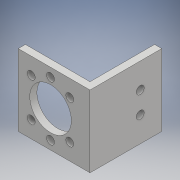
# Autodesk Inventor part: LBent_PScrew
Saved by Autodesk Inventor 2017 (Build 210142000, 142)
## iProperties
Created: 2017-03-12
Part Number: LBent_PScrew
Material: Generic
Document SubType Name: Modeling
Designer: umr
Density: 1 g/cm^3
Appearance: Default
Author: umr
Autodesk Inventor part; units mm, degrees
ref_plane "YZ Plane" through (0, 0, 0) normal (1, 0, 0) x (0, 1, 0)
ref_plane "XZ Plane" through (0, 0, 0) normal (0, 1, 0) x (-1, 0, 0)
ref_plane "XY Plane" through (0, 0, 0) normal (0, 0, 1) x (1, 0, 0)
sketch "Sketch1" plane through (0, 0, 0) normal (0, 0, 1) x (1, 0, 0)
  line L0 (0, 0) -> (-5, 0)
  line L1 (-5, 5) -> (-5, 50)
  line L2 (-5, 50) -> (0, 50)
  line L3 (0, 50) -> (0, 0)
  line L4 (0, 0) -> (-50, 0)
  line L5 (-50, 0) -> (-50, 5)
  line L6 (-50, 5) -> (-5, 5)
  line L7 (0, 5) -> (0, 0)
  dimension "d0" = 5
  dimension "d1" = 50
  dimension "d2" = 50
  dimension "d3" = 5
  constraints: 16 end point, 4 parallel, 2 horizontal, 2 perpendicular
  measures "d0" distance of L1.end L2.end
  measures "d1" distance of L0.end L1.end
  measures "d2" distance of L5.end L7.start
  measures "d3" distance of L4.end L5.end
extrude "Extrusion1" add sketch "Sketch1" along normal blind 50
sketch "Sketch3" plane through (-50, 5, 0) normal (0, 1, 0) x (1, 0, 0)
  circle A0 centre (22.5, -25) radius 14.5
  line L0 (45, 0) -> (0, 0) projected
  line L1 (0, 0) -> (0, -50) projected
  line L2 (45, -50) -> (0, -50) projected
  line L3 (45, 0) -> (45, -50) projected
  line L4 (22.5, -25) -> (0, -25)
  line L5 (22.5, -25) -> (22.5, 0)
  line L6 (45, 0) -> (0, 0) projected
  circle A1 centre (35.935, -38.435) radius 2.75
  circle A2 centre (9.065, -38.435) radius 2.75
  circle A3 centre (22.5, -44) radius 2.75
  circle A4 centre (35.935, -11.565) radius 2.75
  circle A5 centre (9.065, -11.565) radius 2.75
  circle A6 centre (22.5, -6) radius 2.75
  point P0 (50, 0)
  dimension "d44" = 29
  dimension "d45" = 45
  dimension "d46" = 22.5
  dimension "d47" = 25
  dimension "d48" = 5.5
  dimension "d49" = 13.435
  dimension "d50" = 13.435
  dimension "d51" = 5.5
  dimension "d52" = 13.435
  dimension "d53" = 13.435
  dimension "d54" = 5.5
  dimension "d55" = 19
  dimension "d56" = 0
  constraints: 7 centre point, 4 end point, 3 symmetric about line, 2 midpoint, 1 perpendicular, 3 other
  measures "d44" diameter of A0
  measures "d45" distance of L0.start L0.end
  measures "d46" distance from line of L1 L4.start
  measures "d47" distance from line of L0 L4.start
  measures "d48" diameter of A1
  measures "d49" horizontal distance of L4.start A1.centre
  measures "d50" distance from line of L5 A1.centre
  measures "d51" diameter of A2
  measures "d52" distance from line of L4 A2.centre
  measures "d53" distance from line of L5 A2.centre
  measures "d54" diameter of A3
  measures "d55" distance of L4.start A3.centre
  measures "d56" horizontal distance of L4.start A3.centre
extrude "Extrusion2" cut sketch "Sketch3" against normal blind 20 contours A0 L4 L5 | L5 L4 A0 | A6 L5 | L5 A6 | A1 | A2 | A3 | A4 | A5
sketch "Sketch4" plane through (-5, 5, 0) normal (-1, 0, 0) x (0, 0, 1)
  circle A0 centre (17.5, 30) radius 2.75
  line L0 (0, 45) -> (0, 0) projected
  line L1 (0, 45) -> (50, 45) projected
  circle A1 centre (32.5, 30) radius 2.75
  point P0 (0, -5)
  dimension "d59" = 5.5
  dimension "d61" = 17.5
  dimension "d64" = 45
  dimension "d65" = 15
  dimension "d68" = 5.5
  dimension "d69" = 15
  dimension "d70" = 15
  dimension "d71" = 50
  constraints: 2 centre point
  measures "d59" diameter of A0
  measures "d61" distance from line of L0 A0.centre
  measures "d64" distance of L0.start L0.end
  measures "d65" distance from line of L1 A0.centre
  measures "d68" diameter of A1
  measures "d69" distance of A0.centre A1.centre
  measures "d70" distance from line of L1 A1.centre
  measures "d71" distance of L0.start L1.end
extrude "Extrusion3" cut sketch "Sketch4" against normal blind 20
equation "\"d2\" = d1"
equation "\"d3\" = d0"
equation "\"d46\" = 0.5 * d45"
equation "\"d50\" = d49"
equation "\"d52\" = d49"
equation "\"d53\" = d52"
equation "\"d61\" = -0.5 * d69 + 0.5 * d71"
equation "\"d65\" = -0.5 * d63 + 0.5 * d64"
equation "\"d70\" = d65"
equation "\"d63\" = 15"
body "Solid1"
